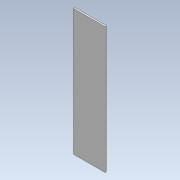
# Autodesk Inventor part: acrylic1
Saved by Autodesk Inventor 2021 (Build 250183000, 183)
## iProperties
Created: 2020-09-26
Part Number: acrylic1
Material: Generic
Document SubType Name: Modeling
Designer: capta
Density: 1 g/cm^3
Appearance: Clear - Blue
Author: capta
Autodesk Inventor part; units mm, degrees
ref_plane "YZ Plane" through (0, 0, 0) normal (1, 0, 0) x (0, 1, 0)
ref_plane "XZ Plane" through (0, 0, 0) normal (0, 1, 0) x (-1, 0, 0)
ref_plane "XY Plane" through (0, 0, 0) normal (0, 0, 1) x (1, 0, 0)
sketch "Sketch1" plane through (0, 0, 0) normal (0, 0, 1) x (1, 0, 0)
  line L0 (-13.6175, 54.61) -> (13.6175, 54.61)
  line L1 (13.6175, 54.61) -> (13.6175, -54.61)
  line L2 (13.6175, -54.61) -> (-13.6175, -54.61)
  line L3 (-13.6175, -54.61) -> (-13.6175, 54.61)
  line L4 (-13.6175, 54.61) -> (13.6175, -54.61) construction
  line L5 (13.6175, 54.61) -> (-13.6175, -54.61) construction
  point P0 (0, 0)
  dimension "d0" = 27.235
  dimension "d1" = 109.22
  constraints: 12 end point, 2 midpoint, 2 parallel, 1 horizontal, 1 perpendicular
  measures "d0" distance of L1.end L2.end
  measures "d1" distance of L0.end L1.end
extrude "Extrusion1" add sketch "Sketch1" along normal blind 1.27
body "Solid1"
